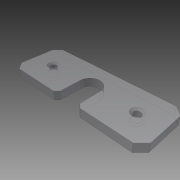
# Autodesk Inventor part: hotend_mount
Saved by Autodesk Inventor 2014 (Build 180170000, 170)
## iProperties
Created: 2013-12-18
Part Number: hotend_mount
Material: Polycarbonate, Clear
Document SubType Name: Modeling
Designer: buben
Density: 1.2 g/cm^3
Appearance: Polycarbonate - Clear
Author: buben
Autodesk Inventor part; units mm, degrees
ref_plane "YZ Plane" through (0, 0, 0) normal (1, 0, 0) x (0, 1, 0)
ref_plane "XZ Plane" through (0, 0, 0) normal (0, 1, 0) x (-1, 0, 0)
ref_plane "XY Plane" through (0, 0, 0) normal (0, 0, 1) x (1, 0, 0)
sketch "Sketch1" plane through (0, 0, 0) normal (0, 0, 1) x (1, 0, 0)
  line L0 (75, 0) -> (75, 27)
  line L1 (75, 27) -> (0, 27)
  line L2 (0, 27) -> (0, 0)
  line L3 (31.5, 0) -> (31.5, 13.5)
  arc A0 (43.5, 13.5) -> (31.5, 13.5) centre (37.5, 13.5) ccw
  line L4 (43.5, 13.5) -> (43.5, 0)
  line L5 (0, 0) -> (31.5, 0)
  line L6 (43.5, 0) -> (75, 0)
  circle A1 centre (12.5, 13.5) radius 2.1
  circle A2 centre (62.5, 13.5) radius 2.1
  point P0 (37.5, 27)
  point P1 (0, 13.5)
  dimension "d0" = 12
  dimension "d1" = 4.2
  dimension "d2" = 50
  dimension "d3" = 25
  dimension "d4" = 75
  dimension "d6" = 13.5
  constraints: 14 end point, 4 parallel, 4 perpendicular, 3 centre point, 3 horizontal alignment, 2 horizontal, 2 midpoint, 2 point on circle, 2 tangent, 1 collinear, 1 equal radius, 1 vertical alignment
  measures "d0" distance between parallel lines of L4 L3
  measures "d1" diameter of A1
  measures "d2" distance of A2.centre A1.centre
  measures "d3" distance of A0.centre A1.centre
  measures "d4" distance between parallel lines of L0 L2
  measures "d6" distance from line of L5 A1.centre
extrude "Extrusion1" add sketch "Sketch1" along normal blind 4.6
chamfer "Chamfer1" distance 4 angle 45 4 edges at (0, 27, 2.3) (0, 0, 2.3) (75, 0, 2.3) (75, 27, 2.3)
chamfer "Chamfer2" distance 2 angle 45 2 edges at (31.5, 0, 2.3) (43.5, 0, 2.3)
chamfer "Chamfer3" distance 1 angle 45 4 edges at (10.4, 13.5, 4.6) (10.4, 13.5, 0) (60.4, 13.5, 0) (60.4, 13.5, 4.6)
equation "\"d3\" = 0.5 * d2"
body "Solid1"
